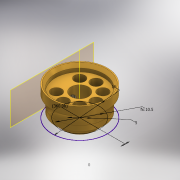
# Autodesk Inventor part: nozzle-base
Saved by Autodesk Inventor 2016 (Build 200138000, 138)
## iProperties
Created: 2015-05-09
Part Number: nozzle-base
Material: Brass, Soft Yellow
Document SubType Name: Modeling
Designer: ax
Mass: 7.2562 g
Surface Area: 11.0977 cm^2
Volume: 0.856694 cm^3
Density: 8.47 g/cm^3
Appearance: Brass - Satin
dO: 16.000 mm
di: 5.000 mm
d2: 10.500 mm
d3: 4,000 ul
d5: 360,00 deg
d7: 8,500 mm
d8: 0,00 deg
dnozzle: 14.000 mm
d10: 2.000 mm
d11: 0,00 deg
d12: 0,700 mm
d13: 1.000 mm
d22: 0,000 mm
d32: -8.000 mm
d33: 3.250 mm
d35: 8.000 mm
d36: 2.459 mm
d41: 8.800 mm
d42: 118,00 deg
deep: 6.500 mm
Author: ax
Autodesk Inventor part; units mm, degrees
ref_plane "XZ Plane" through (0, 0, 0) normal (0, 1, 0) x (-1, 0, 0)
ref_plane "XY Plane" through (0, 0, 0) normal (0, 0, 1) x (1, 0, 0)
sketch "Sketch1" plane through (0, 0, 0) normal (0, 0, 1) x (1, 0, 0)
  circle A0 centre (0, 0) radius 8
  circle A1 centre (0, 0) radius 2.5
  circle A2 centre (0, 0) radius 5.25 construction
  circle A3 centre (0, 0) radius 5.25 construction
  circle A4 centre (0, 0) radius 5.25 construction
  circle A5 centre (0, 0) radius 5.25 construction
  point P0 (-5.25, 0)
  point P1 (0, -5.25)
  point P2 (5.25, 0)
  point P3 (0, 5.25)
  dimension "d2" = 10.5
  dimension "dO" = 16
  dimension "di" = 5
  dimension "d5" = 360
  dimension "d22" = 0
  constraints: 5 coincident, 2 centre point, 2 horizontal alignment, 2 vertical alignment, 19 other
  measures "dO" diameter of A0
  measures "di" diameter of A1
  measures "d22" vertical distance of point (0, 0) point (-5.25, 0)
extrude "Extrusion1" add sketch "Sketch1" along normal blind 8.5
sketch "Sketch2" plane through (0, 0, 8.5) normal (0, 0, 1) x (1, 0, 0)
  circle A0 centre (0, 0) radius 7
  dimension "dnozzle" = 14
  constraints: 1 centre point, 1 coincident
  measures "dnozzle" diameter of A0
extrude "Extrusion2" cut sketch "Sketch2" against normal blind 2
chamfer "Chamfer1" distance 0.7 distance2 1 1 edges at (-7, 0, 8.5) measured on face at (-7.5, 0, 8.5)
ref_plane "Work Plane2" through (-8, 0, 0) normal (1, 0, 0) x (0, 1, 0)
sketch "Sketch5" plane through (-8, 0, 0) normal (1, 0, 0) x (0, 1, 0)
  line L0 (-8, 0) -> (8, 0) projected
  point P0 (0, 0)
  point P1 (0, 3.25)
  dimension "d33" = 3.25
  dimension "d35" = 8
  measures "d33" distance from line of L0 point (0, 3.25)
  measures "d35" horizontal distance of L0.end point (0, 3.25)
hole "Hole3" at (-8, 0, 3.25) direction (1, 0, 0) diameter 2.459 depth 8.8 tip angle 118 thread size "M3x0.5" class "6H" standard "ISO Metric profile"
extrude "Extrusion3" add sketch "Sketch1" against normal blind 1
sketch "Sketch6" plane through (0, 0, 6.5) normal (0, 0, 1) x (1, 0, 0)
  circle A0 centre (0, 0) radius 4.75
  line L0 (0, 0) -> (-14, -14) construction
  point P0 (-3.3588, -3.3588)
  dimension "d48" = 9.5
  constraints: 2 end point, 1 coincident, 1 point on line, 3 other
hole "Hole4" at (-3.3588, -3.3588, 6.5) direction (0, 0, -1) diameter 3 depth 3.1
pattern_circular "Circular Pattern1" count 4 over 360 about axis through (0, 0, 0) along (0, 0, 1) of "Hole4"
pattern_circular "Circular Pattern2" count 2 over 45 about axis through (0, 0, 0) along (0, 0, 1) of "Hole4"
pattern_circular "Circular Pattern3" count 2 over 135 about axis through (0, 0, 0) along (0, 0, 1) of "Hole4"
pattern_circular "Circular Pattern4" count 2 over 225 about axis through (0, 0, 0) along (0, 0, 1) of "Hole4"
sketch "Sketch7" plane through (0, 0, -1) normal (0, 0, -1) x (-1, 0, 0)
  circle A0 centre (0, 0) radius 7
  circle A1 centre (0, 0) radius 8 projected
  dimension "d69" = 14
  constraints: 1 centre point, 1 coincident
  measures "d69" diameter of A0
extrude "Extrusion4" cut sketch "Sketch7" against normal blind 7
fillet "Fillet1" radius 5 1 edges at (7, 0, 6)
chamfer "Chamfer3" distance 2.5 angle 45 1 edges at (7, 0, -1)
equation "\"d2\" = 0.5 * dO + 0.5 * di"
equation "\"d33\" = -0.5 * d10 + 0.5 * d7"
equation "\"d35\" = 0.5 * dO"
equation "\"d32\" = -0.5 * dO"
equation "\"deep\" = d7 - d10"
equation "\"d7\" = 8.5"
equation "\"d10\" = 2"
body "Solid1"
